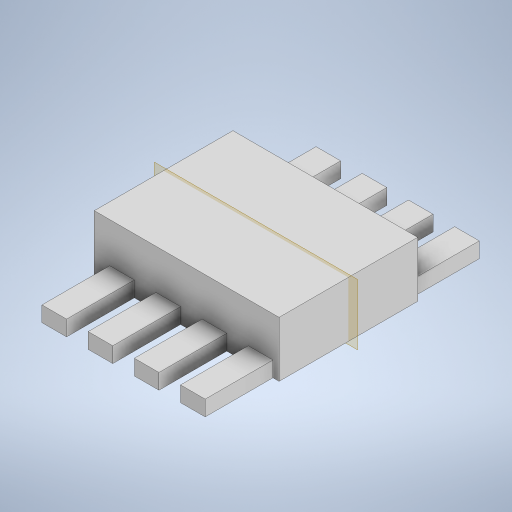
# Autodesk Inventor part: 鏡射
Saved by Autodesk Inventor 2024.2 (Build 282272000, 272)
## iProperties
Created: 2024-05-02
Part Number: 鏡射
Material: 一般
Document SubType Name: Modeling
Designer: User
Density: 1 g/cm^3
Appearance: 預設
Author: User
Autodesk Inventor part; units mm, degrees
ref_plane "YZ Plane" through (0, 0, 0) normal (1, 0, 0) x (0, 1, 0)
ref_plane "XZ Plane" through (0, 0, 0) normal (0, 1, 0) x (-1, 0, 0)
ref_plane "XY Plane" through (0, 0, 0) normal (0, 0, 1) x (1, 0, 0)
sketch "草圖1" plane through (0, 0, 0) normal (0, 1, 0) x (-1, 0, 0)
  line L0 (3, 2.25) -> (-3, 2.25)
  line L1 (-3, 2.25) -> (-3, -2.25)
  line L2 (-3, -2.25) -> (3, -2.25)
  line L3 (3, -2.25) -> (3, 2.25)
  line L4 (3, 2.25) -> (-3, -2.25) construction
  line L5 (-3, 2.25) -> (3, -2.25) construction
  point P0 (0, 0)
  dimension "d0" = 6
  dimension "d1" = 4.5
  constraints: 12 end point, 2 midpoint, 2 parallel, 1 horizontal, 1 perpendicular
  measures "d0" distance of L2.end L1.end
  measures "d1" distance of L0.end L1.end
extrude "擠出1" add sketch "草圖1" along normal blind 1.8
sketch "草圖2" plane through (-3, 0, 2.25) normal (0, 0, 1) x (1, 0, 0)
  line L0 (6, 0) -> (0, 0) projected
  line L1 (0, 0) -> (0.5, 0)
  line L2 (0.5, 0) -> (1.3, 0)
  line L3 (1.3, 0) -> (1.3, 0.5)
  line L4 (1.3, 0.5) -> (0.5, 0.5)
  line L5 (0.5, 0.5) -> (0.5, 0)
  point P0 (3, 0)
  point P1 (1.3, 0)
  dimension "d4" = 0.5
  dimension "d5" = 0.8
  dimension "d6" = 0.5
  constraints: 10 end point, 2 parallel, 1 horizontal, 1 perpendicular, 1 point on line
  measures "d4" distance of L0.end L1.end
  measures "d5" distance of L4.end L3.end
  measures "d6" distance of L3.end L2.end
extrude "擠出2" add sketch "草圖2" along normal blind 2.2
pattern_linear "矩形陣列1" count 4 spacing 1.5 along (1, 0, 0) of "擠出2"
mirror "鏡射1" about plane through (0, 0, 0) normal (0, 0, 1) of "擠出2", "矩形陣列1"
ref_plane "工作平面1" through (-3, 1.8, 0) normal (0, 0, 1) x (1, 0, 0)
